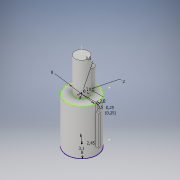
# Autodesk Inventor part: kolo
Saved by Autodesk Inventor 2019 (Build 230136000, 136)
## iProperties
Created: 2020-07-23
Part Number: kolo
Material: Generic
Document SubType Name: Modeling
Designer: lukad
Density: 1 g/cm^3
Appearance: Default
Author: lukad
Autodesk Inventor part; units mm, degrees
ref_plane "YZ Plane" through (0, 0, 0) normal (1, 0, 0) x (0, 1, 0)
ref_plane "XZ Plane" through (0, 0, 0) normal (0, 1, 0) x (-1, 0, 0)
ref_plane "XY Plane" through (0, 0, 0) normal (0, 0, 1) x (1, 0, 0)
sketch "Sketch1" plane through (0, 0, 0) normal (0, 1, 0) x (-1, 0, 0)
  circle A0 centre (2.1789, 5.1456) radius 4
  circle A1 centre (2.1789, 2.9456) radius 1
  circle A2 centre (2.1789, 5.1456) radius 1.75
  point P0 (0, 0)
  dimension "d0" = 8
  dimension "d1" = 2
  dimension "d3" = 3.5
  dimension "d4" = 0
  dimension "d5" = 0
  dimension "d6" = 0
  dimension "d17" = 2.2
  constraints: 3 centre point
  measures "d0" diameter of A0
  measures "d1" diameter of A1
  measures "d3" diameter of A2
  measures "d4" distance of A0.centre A2.centre
  measures "d5" distance of A0.centre A2.centre
  measures "d6" horizontal distance of A0.centre A1.centre
  measures "d17" distance of A1.centre A0.centre
extrude "Extrusion1" add sketch "Sketch1" against normal blind 3 contours A0 | A1 A2 | A2 A1 | A1 A2
extrude "Extrusion2" add sketch "Sketch1" along normal blind 5.4 contours A1 A2 | A2 A1 picked at (1.7556, 3.0976) picked at (2.385, 3.5861)
extrude "Extrusion3" add sketch "Sketch1" along normal blind 9 and the other way blind 12 contours A2 A1 | A1 A2 picked at (2.385, 3.5861) picked at (2.2193, 5.9034)
sketch "Sketch2" plane through (-2.1789, -12, 5.1456) normal (0, -1, 0) x (1, 0, 0)
  circle A0 centre (0, 0) radius 4
  circle A1 centre (0, 0) radius 1.55
  line L0 (-1.2619, 0.9) -> (1.2619, 0.9)
  circle A2 centre (0, 0) radius 4 projected
  point P0 (2.1789, -5.1456)
  dimension "d18" = 8
  dimension "d19" = 3.1
  dimension "d20" = 2.45
  constraints: 2 centre point, 2 end point, 2 point on circle, 1 coincident, 1 concentric, 1 horizontal
  measures "d18" diameter of A0
  measures "d19" diameter of A1
extrude "Extrusion4" add sketch "Sketch2" against normal blind 9 contours A0 | A1 L0 | L0 A1
extrude "Extrusion5" cut sketch "Sketch2" against normal blind 6.2 contours A1 L0 picked at (-0.0386, 0.0848)
sketch "Sketch3" plane through (-2.1789, 0, 5.1456) normal (0, 1, 0) x (1, 0, 0)
  line L0 (3.7119, 0.25) -> (4.7119, 0.25)
  line L1 (4.7119, 0.25) -> (4.7119, -0.25)
  line L2 (4.7119, -0.25) -> (3.7119, -0.25)
  line L3 (3.7119, -0.25) -> (3.7119, 0.25)
  circle A0 centre (0, 0) radius 4 projected
  point P0 (2.1789, 5.1456)
  dimension "d25" = 0.5
  dimension "d26" = 0.25
  dimension "d27" = 0.25
  dimension "d30" = 1
  constraints: 8 end point, 2 parallel, 1 horizontal, 1 perpendicular
  measures "d25" distance between parallel lines of L2 L0
  measures "d26" distance from line of A0.centre L0
  measures "d27" distance from line of A0.centre L2
  measures "d30" distance between parallel lines of L1 L3
extrude "Extrusion6" add sketch "Sketch3" against normal blind 10 contours L0 A0 L2 L3 | L0 L1 L2 A0 picked at (3.8079, 0)
sketch "Sketch4" plane through (0, 0, 0) normal (0, 1, 0) x (1, 0, 0)
  line L0 (1.8133, -4.8956) -> (2.5329, -4.8956) projected
  line L1 (2.5329, -5.3956) -> (1.8133, -5.3956) projected
  line L2 (2.5329, -4.8956) -> (1.8133, -4.8956)
  line L3 (1.8133, -4.8956) -> (1.8133, -5.3956)
  line L4 (1.8133, -5.3956) -> (2.5329, -5.3956)
  line L5 (2.5329, -5.3956) -> (2.5329, -4.8956)
  point P0 (0, 0)
  constraints: 8 end point, 2 parallel, 1 horizontal, 1 perpendicular
extrude "Extrusion7" cut sketch "Sketch4" against normal blind 2
body "Solid1"
